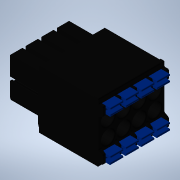
# Autodesk Inventor part: 8079513 8GD-2RR3,5-CLP-CBL
Saved by Autodesk Inventor 2021 (Build 250183000, 183)
## iProperties
Created: 2026-04-23
Part Number: 8079513 8GD-2RR3,5-CLP-CBL
Material: Generic
Catalog Web Link: www.3dfindit.com
Description: NEKM-C6 (p)-terminal strip
Vendor: FESTO
Document SubType Name: Modeling
Designer: psAdmin
Manufacturer: FESTO
Mass: 3.10313 g
Surface Area: 24.1375 cm^2
Volume: 3.10313 cm^3
Density: 1 g/cm^3
Appearance: PSOLRGB-80-80-80
Category: PARTsolutions
Company: FESTO
Title: 8079513 8GD-2RR3,5-CLP-CBL
Author: Cadenas PARTsolutions
Comments: terminal strip
PSOL_IDENT_0: {$CADENAS_DATA/23d-libs/festo/parts/n/nekm/parts/nekm_c6_parts.prj},198 {VTYP=3D},{NB=8079513 8GD-2R
PSOL_IDENT_1: R3,5-CLP-CBL},{LINA=8079513 8GD-2RR3,5-CLP-CBL},{NN=NEKM-C6 (p)},{DATE=26.08.2025 07:05:50},{GEOMDAT
PSOL_IDENT_2: E=26.08.2025 07:05:00},{VERSION=},{LINEID=130},{WBVAR=},{WBNUMERIC=}  {NB=8079513 8GD-2RR3,5-CLP-CBL
PSOL_IDENT_3: },{LINA=8079513 8GD-2RR3,5-CLP-CBL},{KT=DUMMY},{TNR=8079513},{TYP=8GD-2RR3,5-CLP-CBL},{VERS=1},{N=4}
PSOL_IDENT_4: ,{L=14.800},{L1=0.000}
NB: 8079513 8GD-2RR3,5-CLP-CBL
NN: NEKM-C6 (p)
NT: terminal strip
NBSYN: $TNR. $TYP.
LINA: 8079513 8GD-2RR3,5-CLP-CBL
CATALOG: Festo
TNR: 8079513
TYP: 8GD-2RR3,5-CLP-CBL
VERS: 1
N: 4
L: 14.8
L1: 0
SUPPLIER: FESTO
ARTICLENO: 8079513 8GD-2RR3,5-CLP-CBL
BOMINFO: 8079513 8GD-2RR3,5-CLP-CBL
CREATOR: CADENAS GmbH
Autodesk Inventor part; units mm, degrees
sketch "Sketch_1" plane through (0, 0, 0) normal (0, 0, 1) x (1, 0, 0)
  line L0 (0, -4.9505) -> (0.2, -5.5)
  line L1 (0.2, -5.5) -> (0.2, -6.5)
  line L2 (0.2, -6.5) -> (13.4, -6.5)
  arc A0 (13.4, -6.5) -> (13.6, -6.3) centre (13.4, -6.3) ccw
  line L3 (13.6, -6.3) -> (13.6, 6.55)
  arc A1 (13.6, 6.55) -> (13.4, 6.75) centre (13.4, 6.55) ccw
  line L4 (13.4, 6.75) -> (12.8, 6.75)
  arc A2 (12.8, 6.75) -> (12.6, 6.55) centre (12.8, 6.55) ccw
  line L5 (12.6, 6.55) -> (12.6, 6.5)
  line L6 (12.6, 6.5) -> (0.2, 6.5)
  line L7 (0.2, 6.5) -> (0.2, 5.5)
  line L8 (0.2, 5.5) -> (0, 4.9505)
  line L9 (0, 4.9505) -> (0, -4.9505)
  constraints: 20 end point, 6 point on circle, 3 centre point
extrude "Extrusion1" add sketch "Sketch_1" along normal mid plane 14.8
sketch "Sketch_2" plane through (0, 0, 7.4) normal (0, 0, 1) x (1, 0, 0)
  line L0 (13.6, 5.85) -> (13.6, 3.0572)
  arc A0 (13.7, 3.2304) -> (13.6, 3.0572) centre (13.8, 3.0572) ccw
  line L1 (13.7, 3.2304) -> (14.5, 3.6923)
  arc A1 (14.5, 3.6923) -> (14.6, 3.8655) centre (14.4, 3.8655) ccw
  line L2 (14.6, 3.8655) -> (14.6, 5.45)
  arc A2 (14.6, 5.45) -> (14.4, 5.65) centre (14.4, 5.45) ccw
  line L3 (14.4, 5.65) -> (13.8, 5.65)
  arc A3 (13.6, 5.85) -> (13.8, 5.65) centre (13.8, 5.85) ccw
  constraints: 8 end point, 8 point on circle, 4 centre point
extrude "Extrusion2" add sketch "Sketch_2" against normal blind 0.625
sketch "Sketch_3" plane through (0, 0, 7.4) normal (0, 0, 1) x (1, 0, 0)
  arc A0 (13.8, -5.65) -> (13.6, -5.85) centre (13.8, -5.85) ccw
  line L0 (13.8, -5.65) -> (14.4, -5.65)
  arc A1 (14.4, -5.65) -> (14.6, -5.45) centre (14.4, -5.45) ccw
  line L1 (14.6, -5.45) -> (14.6, -3.8655)
  arc A2 (14.6, -3.8655) -> (14.5, -3.6923) centre (14.4, -3.8655) ccw
  line L2 (14.5, -3.6923) -> (13.7, -3.2304)
  arc A3 (13.6, -3.0572) -> (13.7, -3.2304) centre (13.8, -3.0572) ccw
  line L3 (13.6, -3.0572) -> (13.6, -5.85)
  constraints: 8 end point, 8 point on circle, 4 centre point
extrude "Extrusion3" add sketch "Sketch_3" against normal blind 0.625
pattern_linear "Rectangular Pattern1" count 2 spacing 14.175 along (0, 0, -1) of "Extrusion2"
pattern_linear "Rectangular Pattern2" count 2 spacing 14.175 along (0, 0, -1) of "Extrusion3"
sketch "Sketch_8" plane through (0, 0, 3.725) normal (0, 0, 1) x (1, 0, 0)
  line L0 (13.6, 5.85) -> (13.6, 3.0572)
  arc A0 (13.7, 3.2304) -> (13.6, 3.0572) centre (13.8, 3.0572) ccw
  line L1 (13.7, 3.2304) -> (14.5, 3.6923)
  arc A1 (14.5, 3.6923) -> (14.6, 3.8655) centre (14.4, 3.8655) ccw
  line L2 (14.6, 3.8655) -> (14.6, 5.45)
  arc A2 (14.6, 5.45) -> (14.4, 5.65) centre (14.4, 5.45) ccw
  line L3 (14.4, 5.65) -> (13.8, 5.65)
  arc A3 (13.6, 5.85) -> (13.8, 5.65) centre (13.8, 5.85) ccw
  constraints: 8 end point, 8 point on circle, 4 centre point
extrude "Extrusion4" add sketch "Sketch_8" against normal blind 0.45
pattern_linear "Rectangular Pattern3" count 3 spacing 3.5 along (0, 0, -1) of "Extrusion4"
sketch "Sketch_10" plane through (0, 0, 3.725) normal (0, 0, 1) x (1, 0, 0)
  arc A0 (13.8, -5.65) -> (13.6, -5.85) centre (13.8, -5.85) ccw
  line L0 (13.8, -5.65) -> (14.4, -5.65)
  arc A1 (14.4, -5.65) -> (14.6, -5.45) centre (14.4, -5.45) ccw
  line L1 (14.6, -5.45) -> (14.6, -3.8655)
  arc A2 (14.6, -3.8655) -> (14.5, -3.6923) centre (14.4, -3.8655) ccw
  line L2 (14.5, -3.6923) -> (13.7, -3.2304)
  arc A3 (13.6, -3.0572) -> (13.7, -3.2304) centre (13.8, -3.0572) ccw
  line L3 (13.6, -3.0572) -> (13.6, -5.85)
  constraints: 8 end point, 8 point on circle, 4 centre point
extrude "Extrusion5" add sketch "Sketch_10" against normal blind 0.45
pattern_linear "Rectangular Pattern4" count 3 spacing 3.5 along (0, 0, -1) of "Extrusion5"
sketch "Sketch_6" plane through (0, 0, 6.675) normal (0, 0, 1) x (1, 0, 0)
  line L0 (13.6, 3.85) -> (15.4, 3.85)
  arc A0 (15.4, 3.85) -> (15.6, 4.05) centre (15.4, 4.05) ccw
  line L1 (15.6, 4.05) -> (15.6, 4.0747)
  arc A1 (15.6, 4.0747) -> (15.4261, 4.273) centre (15.4, 4.0747) ccw
  line L2 (15.4261, 4.273) -> (14.4418, 4.4026)
  arc A2 (14.4418, 4.9974) -> (14.4418, 4.4026) centre (14.481, 4.7) ccw
  line L3 (14.4418, 4.9974) -> (15.4261, 5.127)
  arc A3 (15.4261, 5.127) -> (15.6, 5.3253) centre (15.4, 5.3253) ccw
  line L4 (15.6, 5.3253) -> (15.6, 5.35)
  arc A4 (15.6, 5.35) -> (15.4, 5.55) centre (15.4, 5.35) ccw
  line L5 (15.4, 5.55) -> (13.6, 5.55)
  line L6 (13.6, 5.55) -> (13.6, 3.85)
  constraints: 14 end point, 10 point on circle, 5 centre point
extrude "Extrusion6" add sketch "Sketch_6" against normal blind 2.85
pattern_linear "Rectangular Pattern5" count 4 spacing 3.5 along (0, 0, -1) count 2 spacing 9.4 along (0, -1, 0) of "Extrusion6"
sketch "Sketch_12" plane through (0, 1.8, 0) normal (0, 1, 0) x (1, 0, 0)
  line L0 (10.6, -5.25) -> (13.6, -5.25)
  line L1 (13.6, -5.25) -> (13.6, -6.95)
  arc A0 (13.6, -6.95) -> (13.4, -6.75) centre (13.4, -6.95) ccw
  line L2 (13.4, -6.75) -> (10.6, -6.75)
  line L3 (10.6, -6.75) -> (10.6, -5.25)
  line L4 (10.6, -5.25) -> (13.6, -5.25)
  constraints: 10 end point, 2 point on circle, 1 centre point
revolve "Revolution1" cut sketch "Sketch_12" angle 360 about axis through (10.6, 1.8, 5.25) along (-1, 0, 0)
pattern_linear "Rectangular Pattern6" count 4 spacing 3.5 along (0, 0, -1) count 2 spacing 3.6 along (0, -1, 0) of "Revolution1"
sketch "Sketch_14" plane through (0, 0, 0) normal (1, 0, 0) x (0, 1, 0)
  line L0 (0.4, 6.625) -> (0.4, 6.2838)
  arc A0 (0.4, 6.2838) -> (0.4586, 6.1424) centre (0.6, 6.2838) ccw
  line L1 (0.4586, 6.1424) -> (0.7278, 5.8732)
  arc A1 (0.8266, 5.527) -> (0.7278, 5.8732) centre (-0.8, 5.25) ccw
  line L2 (0.8266, 5.527) -> (0.6203, 5.3207)
  arc A2 (0.6203, 5.3207) -> (0.6203, 5.1793) centre (0.691, 5.25) ccw
  line L3 (0.6203, 5.1793) -> (0.8266, 4.973)
  arc A3 (0.7278, 4.6268) -> (0.8266, 4.973) centre (-0.8, 5.25) ccw
  line L4 (0.7278, 4.6268) -> (0.4586, 4.3576)
  arc A4 (0.4586, 4.3576) -> (0.4, 4.2162) centre (0.6, 4.2162) ccw
  line L5 (0.4, 4.2162) -> (0.4, 3.875)
  line L6 (0.4, 3.875) -> (4.6, 3.875)
  line L7 (4.6, 3.875) -> (4.6, 6.625)
  line L8 (4.6, 6.625) -> (0.4, 6.625)
  constraints: 18 end point, 10 point on circle, 5 centre point
extrude "Extrusion7" add sketch "Sketch_14" against normal blind 7.05
pattern_linear "Rectangular Pattern7" count 4 spacing 3.5 along (0, 0, -1) of "Extrusion7"
sketch "Sketch_16" plane through (0, 0, 0) normal (1, 0, 0) x (0, 1, 0)
  arc A0 (-3.6989, 6.625) -> (-4.6, 5.7239) centre (-3.6989, 5.7239) ccw
  line L0 (-4.6, 5.7239) -> (-4.6, 4.7761)
  arc A1 (-4.6, 4.7761) -> (-3.6989, 3.875) centre (-3.6989, 4.7761) ccw
  line L1 (-3.6989, 3.875) -> (-0.4, 3.875)
  line L2 (-0.4, 3.875) -> (-0.4, 4.2162)
  arc A2 (-0.4, 4.2162) -> (-0.4586, 4.3576) centre (-0.6, 4.2162) ccw
  line L3 (-0.4586, 4.3576) -> (-0.7278, 4.6268)
  arc A3 (-0.8266, 4.973) -> (-0.7278, 4.6268) centre (0.8, 5.25) ccw
  line L4 (-0.8266, 4.973) -> (-0.6203, 5.1793)
  arc A4 (-0.6203, 5.1793) -> (-0.6203, 5.3207) centre (-0.691, 5.25) ccw
  line L5 (-0.6203, 5.3207) -> (-0.8266, 5.527)
  arc A5 (-0.7278, 5.8732) -> (-0.8266, 5.527) centre (0.8, 5.25) ccw
  line L6 (-0.7278, 5.8732) -> (-0.4586, 6.1424)
  arc A6 (-0.4586, 6.1424) -> (-0.4, 6.2838) centre (-0.6, 6.2838) ccw
  line L7 (-0.4, 6.2838) -> (-0.4, 6.625)
  line L8 (-0.4, 6.625) -> (-3.6989, 6.625)
  constraints: 18 end point, 14 point on circle, 7 centre point
extrude "Extrusion8" add sketch "Sketch_16" against normal blind 7.05
pattern_linear "Rectangular Pattern8" count 4 spacing 3.5 along (0, 0, -1) of "Extrusion8"
sketch "Sketch_18" plane through (0, 2.75, 0) normal (0, 1, 0) x (1, 0, 0)
  line L0 (-6.05, -5.25) -> (-7.05, -5.25)
  line L1 (-7.05, -5.25) -> (-7.05, -4.45)
  line L2 (-7.05, -4.45) -> (-6.05, -4.45)
  line L3 (-6.05, -4.45) -> (-6.05, -5.25)
  line L4 (-6.05, -5.25) -> (-7.05, -5.25)
  constraints: 10 end point
revolve "Revolution2" cut sketch "Sketch_18" angle 360 about axis through (-6.05, 2.75, 5.25) along (1, 0, 0)
pattern_linear "Rectangular Pattern9" count 4 spacing 3.5 along (0, 0, -1) count 2 spacing 5.5 along (0, -1, 0) of "Revolution2"
ref_plane "ANBAU_XY" through (0, 0, 0) normal (0, 1, 0) x (1, 0, 0)
ref_plane "ANBAU_YZ" through (0, 0, 0) normal (1, 0, 0) x (0, 0, -1)
ref_plane "ANBAU_ZX" through (0, 0, 0) normal (0, 0, -1) x (0, 1, 0)
ref_plane "CP1_XY" through (0, 0, 0) normal (1, 0, 0) x (0, 0, -1)
ref_plane "CP1_YZ" through (0, 0, 0) normal (0, 0, -1) x (0, 1, 0)
ref_plane "CP1_ZX" through (0, 0, 0) normal (0, 1, 0) x (1, 0, 0)
ref_plane "ECP_1_XY" through (2.6, 1.8, 5.25) normal (1, 0, 0) x (0, 0, -1)
ref_plane "ECP_1_YZ" through (2.6, 1.8, 5.25) normal (0, 0, -1) x (0, 1, 0)
ref_plane "ECP_1_ZX" through (2.6, 1.8, 5.25) normal (0, 1, 0) x (1, 0, 0)
ref_plane "ECP_2_XY" through (2.6, 1.8, 1.75) normal (1, 0, 0) x (0, 0, -1)
ref_plane "ECP_2_YZ" through (2.6, 1.8, 1.75) normal (0, 0, -1) x (0, 1, 0)
ref_plane "ECP_2_ZX" through (2.6, 1.8, 1.75) normal (0, 1, 0) x (1, 0, 0)
ref_plane "ECP_3_XY" through (2.6, 1.8, -1.75) normal (1, 0, 0) x (0, 0, -1)
ref_plane "ECP_3_YZ" through (2.6, 1.8, -1.75) normal (0, 0, -1) x (0, 1, 0)
ref_plane "ECP_3_ZX" through (2.6, 1.8, -1.75) normal (0, 1, 0) x (1, 0, 0)
ref_plane "ECP_4_XY" through (2.6, 1.8, -5.25) normal (1, 0, 0) x (0, 0, -1)
ref_plane "ECP_4_YZ" through (2.6, 1.8, -5.25) normal (0, 0, -1) x (0, 1, 0)
ref_plane "ECP_4_ZX" through (2.6, 1.8, -5.25) normal (0, 1, 0) x (1, 0, 0)
ref_plane "ECP_5_XY" through (2.6, -1.8, 5.25) normal (1, 0, 0) x (0, 0, -1)
ref_plane "ECP_5_YZ" through (2.6, -1.8, 5.25) normal (0, 0, -1) x (0, 1, 0)
ref_plane "ECP_5_ZX" through (2.6, -1.8, 5.25) normal (0, 1, 0) x (1, 0, 0)
ref_plane "ECP_6_XY" through (2.6, -1.8, 1.75) normal (1, 0, 0) x (0, 0, -1)
ref_plane "ECP_6_YZ" through (2.6, -1.8, 1.75) normal (0, 0, -1) x (0, 1, 0)
ref_plane "ECP_6_ZX" through (2.6, -1.8, 1.75) normal (0, 1, 0) x (1, 0, 0)
ref_plane "ECP_7_XY" through (2.6, -1.8, -1.75) normal (1, 0, 0) x (0, 0, -1)
ref_plane "ECP_7_YZ" through (2.6, -1.8, -1.75) normal (0, 0, -1) x (0, 1, 0)
ref_plane "ECP_7_ZX" through (2.6, -1.8, -1.75) normal (0, 1, 0) x (1, 0, 0)
ref_plane "ECP_8_XY" through (2.6, -1.8, -5.25) normal (1, 0, 0) x (0, 0, -1)
ref_plane "ECP_8_YZ" through (2.6, -1.8, -5.25) normal (0, 0, -1) x (0, 1, 0)
ref_plane "ECP_8_ZX" through (2.6, -1.8, -5.25) normal (0, 1, 0) x (1, 0, 0)
ref_plane "MD_XY" through (-7.05, 2.75, 5.25) normal (-1, 0, 0) x (0, 0, -1)
ref_plane "MD_YZ" through (-7.05, 2.75, 5.25) normal (0, 0, -1) x (0, -1, 0)
ref_plane "MD_ZX" through (-7.05, 2.75, 5.25) normal (0, -1, 0) x (-1, 0, 0)
ref_plane "OP_XY" through (-7.05, 6.625, -7.4) normal (1, 0, 0) x (0, 0, 1)
ref_plane "OP_YZ" through (-7.05, 6.625, -7.4) normal (0, 0, 1) x (0, -1, 0)
ref_plane "OP_ZX" through (-7.05, 6.625, -7.4) normal (0, -1, 0) x (1, 0, 0)
body "Solid1"
